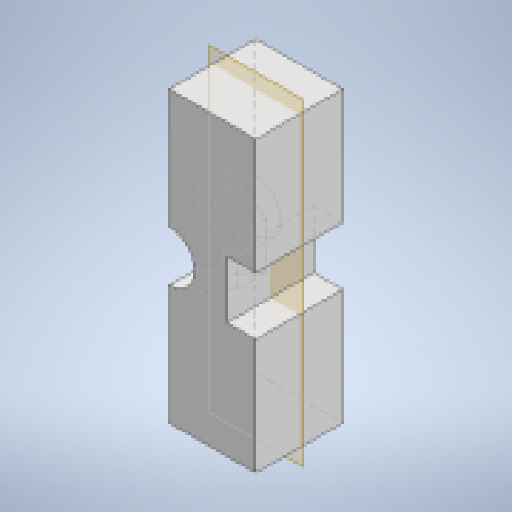
# Autodesk Inventor part: POMSliderMotor
Saved by Autodesk Inventor 2023 (Build 270158000, 158)
## iProperties
Created: 2023-03-27
Part Number: POMSliderMotor
Material: Generic
Document SubType Name: Modeling
Designer: Nathann
Density: 1 g/cm^3
Appearance: Default
Author: Nathann
Autodesk Inventor part; units mm, degrees
ref_plane "YZ Plane" through (0, 0, 0) normal (1, 0, 0) x (0, 1, 0)
ref_plane "XZ Plane" through (0, 0, 0) normal (0, 1, 0) x (-1, 0, 0)
ref_plane "XY Plane" through (0, 0, 0) normal (0, 0, 1) x (1, 0, 0)
sketch "Sketch1" plane through (0, 0, 0) normal (0, 0, 1) x (1, 0, 0)
  line L0 (10, -10) -> (-10, -10)
  line L1 (-10, -10) -> (-10, 10)
  line L2 (-10, 10) -> (10, 10)
  line L3 (10, 10) -> (10, -10)
  line L4 (10, -10) -> (-10, 10) construction
  line L5 (-10, -10) -> (10, 10) construction
  line L6 (10, -10) -> (6, -10)
  line L7 (6, -10) -> (6, 10)
  line L8 (6, 10) -> (10, 10)
  line L9 (10, 10) -> (10, -10)
  line L10 (6, 2) -> (4, 2)
  line L11 (4, 2) -> (4, -2)
  line L12 (4, -2) -> (6, -2)
  line L13 (6, -2) -> (6, 2)
  line L14 (0, 10) -> (0, -10)
  point P0 (0, 0)
  dimension "d0" = 20
  dimension "d1" = 20
  dimension "d2" = 4
  dimension "d6" = 2
  dimension "d7" = 2
  dimension "d8" = 4
  dimension "d9" = 2
  constraints: 30 end point, 6 parallel, 4 midpoint, 3 horizontal, 3 perpendicular, 3 point on line
  measures "d0" distance of L1.end L2.end
  measures "d1" distance of L0.end L1.end
  measures "d2" distance between parallel lines of L3 L7
  measures "d6" distance from line of L10 point (0, 0)
  measures "d7" distance from line of L12 point (0, 0)
  measures "d8" distance of L10.end L11.end
  measures "d9" distance of L10.start L10.end
extrude "Extrusion1" add sketch "Sketch1" along normal blind 5 contours L0 L14 L2 L7 L10 L11 L12
ref_plane "Work Plane1" through (0, 0, 2.5) normal (0, 0, 1) x (1, 0, 0)
sketch "Sketch2" plane through (0, 0, 2.5) normal (0, 0, 1) x (1, 0, 0)
  line L0 (0, 10) -> (0, -10) projected
  line L1 (0, 3.1754) -> (2.75, 1.5877)
  line L2 (2.75, 1.5877) -> (2.75, -1.5877)
  line L3 (2.75, -1.5877) -> (0, -3.1754)
  line L4 (0, -3.1754) -> (-2.75, -1.5877)
  line L5 (-2.75, -1.5877) -> (-2.75, 1.5877)
  line L6 (-2.75, 1.5877) -> (0, 3.1754)
  point P0 (0, 0)
  point P1 (0, 0)
  dimension "d12" = 5.5
  constraints: 12 end point, 1 coincident, 1 point on line, 13 other
  measures "d12" distance between parallel lines of L2 L5
extrude "Extrusion2" cut sketch "Sketch2" along normal mid plane 1.8
sketch "Sketch3" plane through (0, 0, 5) normal (0, 0, 1) x (1, 0, 0)
  circle A0 centre (0, 0) radius 1.75
  dimension "d15" = 3.5
  constraints: 1 centre point, 1 coincident
  measures "d15" diameter of A0
extrude "Extrusion3" cut sketch "Sketch3" against normal blind 8
body "Solid1"
